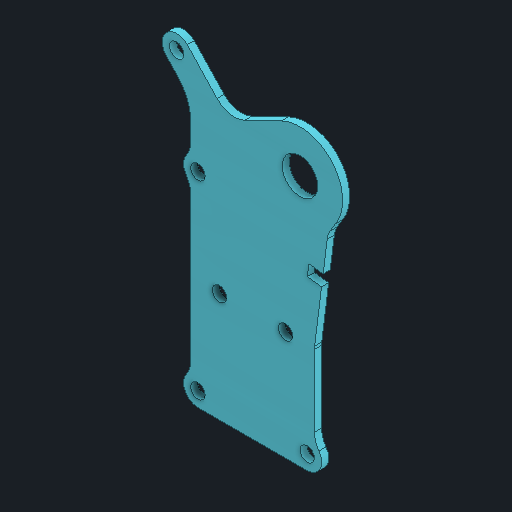
# Autodesk Inventor part: tibea_outside_steel
Saved by Autodesk Inventor 2026 (Build 300175000, 175)
## iProperties
Created: 2026-04-23
Part Number: tibea_outside_steel
Material: Сталь
Document SubType Name: Modeling
Designer: user
Density: 7.85 g/cm^3
Appearance: Серо-синий
Mass: 154.038 g
Surface Area: 147.821 cm^2
Volume: 19.6226 cm^3
Author: user
Autodesk Inventor part; units mm, degrees
ref_plane "YZ Plane" through (0, 0, 0) normal (1, 0, 0) x (0, 1, 0)
ref_plane "XZ Plane" through (0, 0, 0) normal (0, 1, 0) x (-1, 0, 0)
ref_plane "XY Plane" through (0, 0, 0) normal (0, 0, 1) x (1, 0, 0)
sketch "Эскиз1" plane through (0, 0, 0) normal (0, 0, 1) x (1, 0, 0)
  line L0 (-302.1837, 10.5492) -> (-302.1837, 99.2824)
  line L1 (-302.1837, 21.7824) -> (-325.2337, 21.7824)
  circle A0 centre (-325.2337, 27.8824) radius 3.05
  arc A1 (-330.1781, 31.4549) -> (-325.2337, 21.7824) centre (-325.2337, 27.8824) ccw
  circle A2 centre (-316.1337, 67.8824) radius 3.05
  line L2 (-328.2837, 37.3115) -> (-328.2837, 98.4533)
  arc A3 (-330.1781, 111.4549) -> (-330.1781, 104.3099) centre (-325.2337, 107.8824) ccw
  circle A4 centre (-325.2337, 107.8824) radius 3.05
  line L3 (-302.1837, 21.7824) -> (-279.1337, 21.7824)
  circle A5 centre (-279.1337, 27.8824) radius 3.05
  arc A6 (-279.1337, 21.7824) -> (-274.1893, 31.4549) centre (-279.1337, 27.8824) ccw
  circle A7 centre (-288.2337, 67.8824) radius 3.05
  line L4 (-276.0837, 37.3115) -> (-276.0837, 67.5687)
  circle A8 centre (-282.1837, 127.8824) radius 7.5
  circle A9 centre (-334.1837, 147.8824) radius 3.05
  arc A10 (-328.2837, 98.4533) -> (-330.1781, 104.3099) centre (-338.2837, 98.4533) ccw
  arc A11 (-276.0837, 37.3115) -> (-274.1893, 31.4549) centre (-266.0837, 37.3115) ccw
  arc A12 (-330.1781, 31.4549) -> (-328.2837, 37.3115) centre (-338.2837, 37.3115) ccw
  arc A13 (-267.2469, 117.838) -> (-290.0489, 144.0731) centre (-282.1837, 127.8824) ccw
  line L5 (-337.6238, 138.6125) -> (-337.5598, 138.5762)
  line L6 (-328.2837, 117.3115) -> (-328.2837, 124.794)
  arc A14 (-330.1781, 111.4549) -> (-328.2837, 117.3115) centre (-338.2837, 117.3115) ccw
  line L7 (-274.7426, 126.9449) -> (-276.7879, 110.7102) construction
  line L8 (-279.0587, 92.6863) -> (-273.093, 91.9347)
  line L9 (-278.4212, 97.7463) -> (-272.4165, 96.9898)
  line L10 (-279.0587, 92.6863) -> (-282.1837, 67.8824) construction
  line L11 (-278.4212, 97.7463) -> (-279.0587, 92.6863)
  line L12 (-276.7879, 110.7102) -> (-278.4212, 97.7463) construction
  arc A15 (-267.2469, 117.838) -> (-269.5554, 114.0527) centre (-225.7555, 89.937) ccw
  line L13 (-276.0053, 68.8187) -> (-273.093, 91.9347)
  line L14 (-272.4165, 96.9898) -> (-270.717, 110.4795)
  arc A16 (-269.5554, 114.0527) -> (-270.717, 110.4795) centre (-260.7954, 109.2295) ccw
  arc A17 (-276.0053, 68.8187) -> (-276.0837, 67.5687) centre (-266.0837, 67.5687) ccw
  line L15 (-334.1836, 156.7715) -> (-317.1375, 138.7027) construction
  arc A18 (-329.7466, 152.0683) -> (-338.6208, 143.6964) centre (-334.1837, 147.8824) ccw
  line L16 (-305.4941, 136.5701) -> (-290.0489, 144.0731)
  line L17 (-317.1375, 138.7027) -> (-329.7466, 152.0683)
  arc A19 (-317.1375, 138.7027) -> (-305.4941, 136.5701) centre (-309.8636, 145.5649) ccw
  line L18 (-338.6208, 143.6964) -> (-333.7359, 138.5184)
  arc A20 (-328.2837, 124.794) -> (-333.7359, 138.5184) centre (-348.2837, 124.794) ccw
  point P0 (-328.2837, 33.1651)
  point P1 (-328.2837, 102.5996)
  point P2 (-276.0837, 33.1651)
  point P3 (-274.7318, 111.4974)
  point P4 (-331.3337, 107.8824)
  point P5 (-276.0837, 110.9475)
  point P6 (-274.8637, 144.3268)
  point P7 (-328.2837, 163.1651)
  point P8 (-291.0588, 112.2224)
  point P9 (-328.2837, 113.1651)
  point P10 (-276.0837, 92.3115)
  point P11 (-275.2043, 97.341)
  point P12 (-276.0087, 92.302)
  point P13 (-270.4917, 112.268)
  dimension "d13" = 15
  dimension "d0" = 6.1
  dimension "d1" = 12.2
  dimension "d2" = 46.1
  dimension "d10" = 80
  dimension "d11" = 40
  dimension "d12" = 9.1
  dimension "d15" = 60
  dimension "d17" = 20
  dimension "d23" = 36
  dimension "d31" = 10
  dimension "d33" = 6.1
  dimension "d35" = 5.1
  dimension "d36" = 25
  dimension "d37" = 50
  dimension "d41" = 18
  dimension "d42" = 12.2
  dimension "d43" = 52
  dimension "d44" = 20
  dimension "d45" = 10
  dimension "d46" = 20
  constraints: 39 point on circle, 38 end point, 23 tangent, 20 centre point, 13 point on line, 9 equal radius, 6 perpendicular, 5 coincident, 5 symmetric about line, 4 vertical, 3 parallel, 2 vertical alignment, 1 horizontal, 1 horizontal alignment, 11 other
  measures "d0" diameter of A0
  measures "d1" diameter of A1
  measures "d2" diameter of A0.centre L0
  measures "d10" distance of A3.centre A0.centre
  measures "d11" vertical distance of A0.centre A2.centre
  measures "d12" horizontal distance of A2.centre A0.centre
  measures "d15" vertical distance of point (-282.184, 127.882) A7.centre
  measures "d17" distance from line of L0 point (-282.184, 127.882)
  measures "d23" diameter of A13
  measures "d31" radius of A14
  measures "d33" distance from line of L10.end L4
  measures "d35" distance from line of L9 point (-276.009, 92.302)
  measures "d36" distance from line of L10.end L8
  measures "d37" radius of A15
  measures "d41" distance from line of point (-282.184, 127.882) L15
  measures "d42" diameter of A18
  measures "d43" horizontal distance of A9.centre point (-282.184, 127.882)
  measures "d44" vertical distance of A9.centre point (-282.184, 127.882)
  measures "d45" radius of A19
  measures "d46" radius of A20
extrude "Выдавливание1" add sketch "Эскиз1" along normal blind 3
equation "\"d13\" = d_main_shaft"
equation "\"d0\" = d_main_screw_holes"
equation "\"d1\" = 2 * d_main_screw_holes"
equation "\"d2\" = hight_profile_tibea + d_main_screw_holes"
equation "\"d12\" = d_main_screw_holes + thickness_profile_tibea"
equation "\"d21\" = thickness_steel"
equation "\"tolerance_plazma\" = 0.1"
equation "\"thickness_steel\" = 3"
equation "\"d_main_screw_holes\" = 6.1"
equation "\"d_main_shaft\" = 15"
equation "\"thickness_profile_tibea\" = 3"
equation "\"hight_profile_tibea\" = 40"
equation "\"hight_shaft_shift\" = 37"
equation "\"thickness_profile_femur\" = 3"
equation "\"width_shaft_shift\" = 35"
equation "\"width_flattened_surface\" = 12"
